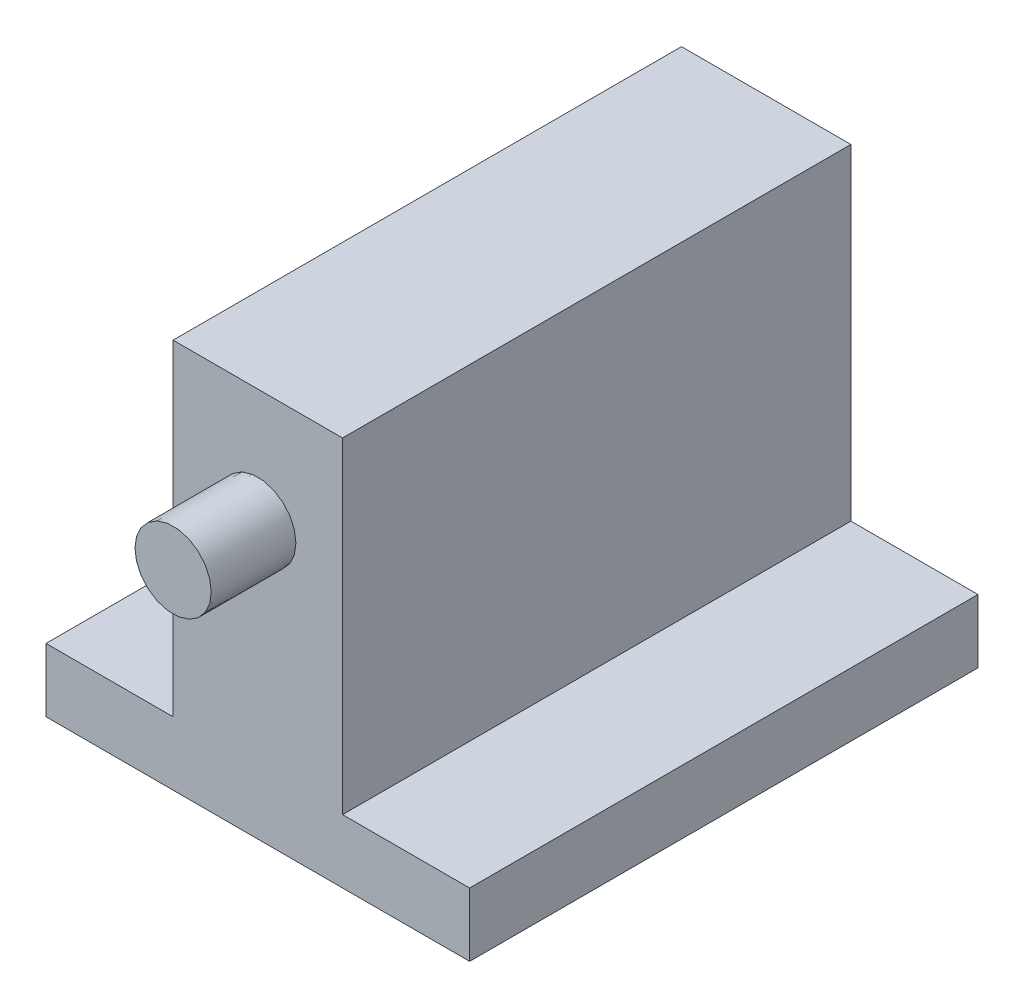
# Autodesk Inventor part: Tailstock
Saved by Autodesk Inventor 2023 (Build 270158000, 158)
## iProperties
Created: 2024-08-24
Part Number: Tailstock
Material: Generic
Document SubType Name: Modeling
Designer: think
Density: 1 g/cm^3
Appearance: Default
Author: think
Autodesk Inventor part; units mm, degrees
ref_plane "YZ Plane" through (0, 0, 0) normal (1, 0, 0) x (0, 1, 0)
ref_plane "XZ Plane" through (0, 0, 0) normal (0, 1, 0) x (-1, 0, 0)
ref_plane "XY Plane" through (0, 0, 0) normal (0, 0, 1) x (1, 0, 0)
sketch "Sketch1" plane through (0, 0, 0) normal (0, 0, 1) x (1, 0, 0)
  line L0 (0, 0) -> (0, 15)
  line L1 (0, 15) -> (30, 15)
  line L2 (30, 15) -> (30, 92)
  line L3 (30, 92) -> (70, 92)
  line L4 (70, 92) -> (70, 15)
  line L5 (70, 15) -> (100, 15)
  line L6 (100, 15) -> (100, 0)
  line L7 (100, 0) -> (0, 0)
  dimension "d0" = 15
  dimension "d1" = 92
  dimension "d2" = 40
  dimension "d3" = 100
  constraints: 16 end point, 6 perpendicular, 2 point on line, 1 collinear, 1 vertical
  measures "d0" distance of L0.start L0.end
  measures "d1" distance from line of L0.start L3
  measures "d2" distance of L2.end L3.end
  measures "d3" distance of L6.end L0.start
extrude "Extrusion1" add sketch "Sketch1" along normal blind 120
sketch "Sketch2" plane through (0, 0, 120) normal (0, 0, 1) x (1, 0, 0)
  circle A0 centre (50, 65) radius 9
  line L0 (0, 0) -> (100, 0) projected
  line L1 (50, 65) -> (50, 0) construction
  line L2 (0, 0) -> (100, 0) construction
  dimension "d6" = 65
  dimension "d7" = 18
  constraints: 2 end point, 1 centre point, 1 midpoint, 1 vertical
  measures "d6" distance of L1.start L1.end
  measures "d7" diameter of A0
extrude "Extrusion2" add sketch "Sketch2" along normal blind 20
body "Solid1"
